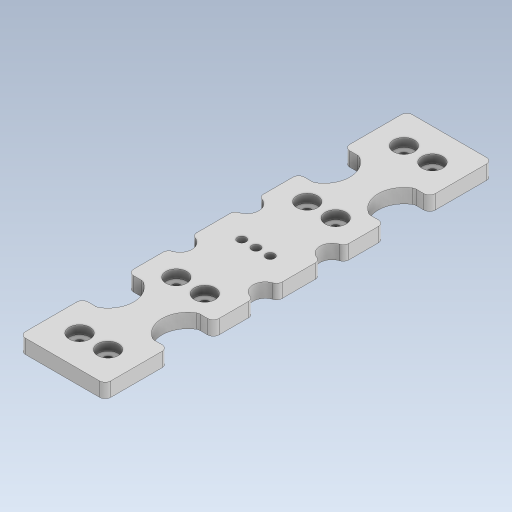
# Autodesk Inventor part: Stopper Lifter
Saved by Autodesk Inventor 2023.5 (Build 275446000, 446)
## iProperties
Created: 2025-10-05
Part Number: Stopper Lifter
Material: Generic
Document SubType Name: Modeling
Designer: Guntur
Density: 1 g/cm^3
Appearance: Default
Author: Guntur
Autodesk Inventor part; units mm, degrees
ref_plane "YZ Plane" through (0, 0, 0) normal (1, 0, 0) x (0, 1, 0)
ref_plane "XZ Plane" through (0, 0, 0) normal (0, 1, 0) x (-1, 0, 0)
ref_plane "XY Plane" through (0, 0, 0) normal (0, 0, 1) x (1, 0, 0)
sketch "Sketch1" plane through (0, 0, 0) normal (0, 1, 0) x (-1, 0, 0)
  line L0 (13.7897, -1.2319) -> (-9.6368, -1.2319) construction
  line L1 (0.7897, 10.3965) -> (0.7897, -17.2319) construction
  line L2 (0.7897, -1.2319) -> (15.7897, -1.2319)
  line L3 (15.7897, -1.2319) -> (15.7897, -7.0606)
  line L4 (15.7897, -8.7319) -> (0.7897, -8.7319)
  line L5 (0.7897, -8.7319) -> (0.7897, -1.2319)
  line L6 (21.7897, -1.2319) -> (-22.2103, -1.2319) construction
  line L7 (0.7897, 17.7681) -> (0.7897, -29.2319) construction
  circle A0 centre (5.7897, -24.2319) radius 3.65
  circle A1 centre (5.7897, -24.2319) radius 5
  circle A2 centre (5.7897, -58.2319) radius 3.65
  circle A3 centre (5.7897, -58.2319) radius 5
  line L8 (0.7897, -17.2319) -> (15.7897, -17.2319)
  line L9 (15.7897, -18.9033) -> (15.7897, -29.2319)
  line L10 (13.7897, -31.2319) -> (11.138, -31.2319)
  line L11 (0.7897, -31.2319) -> (0.7897, -17.2319)
  line L12 (0.7897, -51.2319) -> (15.7897, -51.2319)
  line L13 (15.7897, -51.2319) -> (15.7897, -65.2319)
  line L14 (15.7897, -65.2319) -> (0.7897, -65.2319)
  line L15 (0.7897, -65.2319) -> (0.7897, -51.2319)
  arc A4 (14.4297, -8.9554) -> (14.4297, -17.0085) centre (15.7897, -12.9819) ccw
  line L16 (15.7897, -51.2319) -> (0.7897, -51.2319)
  line L17 (0.7897, -51.2319) -> (0.7897, -47.2319)
  line L18 (11.138, -47.2319) -> (13.7897, -47.2319)
  line L19 (15.7897, -49.2319) -> (15.7897, -51.2319)
  line L20 (15.7897, -65.2319) -> (0.7897, -65.2319)
  line L21 (0.7897, -65.2319) -> (0.7897, -69.2319)
  line L22 (0.7897, -69.2319) -> (13.7897, -69.2319)
  line L23 (15.7897, -67.2319) -> (15.7897, -65.2319)
  arc A5 (14.4297, -8.9554) -> (15.7897, -7.0606) centre (13.7897, -7.0606) ccw
  arc A6 (15.7897, -18.9033) -> (14.4297, -17.0085) centre (13.7897, -18.9033) ccw
  arc A7 (-12.8503, -17.0085) -> (-14.2103, -18.9033) centre (-12.2103, -18.9033) ccw
  circle A8 centre (-4.2103, -24.2319) radius 3.65
  circle A9 centre (-4.2103, -24.2319) radius 5
  line L24 (0.7897, -17.2319) -> (-14.2103, -17.2319)
  arc A10 (-12.8503, -17.0085) -> (-12.8503, -8.9554) centre (-14.2103, -12.9819) ccw
  arc A11 (-14.2103, -7.0606) -> (-12.8503, -8.9554) centre (-12.2103, -7.0606) ccw
  line L25 (-14.2103, -8.7319) -> (0.7897, -8.7319)
  line L26 (-14.2103, -1.2319) -> (-14.2103, -7.0606)
  line L27 (-14.2103, -18.9033) -> (-14.2103, -29.2319)
  line L28 (-12.2103, -31.2319) -> (-9.5586, -31.2319)
  line L29 (-14.2103, -49.2319) -> (-14.2103, -51.2319)
  line L30 (-9.5586, -47.2319) -> (-12.2103, -47.2319)
  line L31 (0.7897, -51.2319) -> (-14.2103, -51.2319)
  line L32 (-14.2103, -51.2319) -> (0.7897, -51.2319)
  line L33 (-14.2103, -51.2319) -> (-14.2103, -65.2319)
  circle A12 centre (-4.2103, -58.2319) radius 3.65
  circle A13 centre (-4.2103, -58.2319) radius 5
  line L34 (-14.2103, -67.2319) -> (-14.2103, -65.2319)
  line L35 (-14.2103, -65.2319) -> (0.7897, -65.2319)
  line L36 (-14.2103, -65.2319) -> (0.7897, -65.2319)
  line L37 (0.7897, -69.2319) -> (-12.2103, -69.2319)
  line L38 (0.7897, 6.2681) -> (0.7897, -1.2319)
  arc A14 (-12.8503, 6.4915) -> (-12.8503, 14.5446) centre (-14.2103, 10.5181) ccw
  line L39 (-14.2103, 6.2681) -> (0.7897, 6.2681)
  line L40 (-14.2103, -1.2319) -> (-14.2103, 4.5967)
  arc A15 (-12.8503, 6.4915) -> (-14.2103, 4.5967) centre (-12.2103, 4.5967) ccw
  line L41 (15.7897, -1.2319) -> (15.7897, 4.5967)
  line L42 (15.7897, 6.2681) -> (0.7897, 6.2681)
  line L43 (0.7897, -12.8604) -> (0.7897, 14.7681) construction
  line L44 (0.7897, -20.2319) -> (0.7897, 26.7681) construction
  circle A16 centre (5.7897, 55.7681) radius 3.65
  circle A17 centre (5.7897, 55.7681) radius 5
  line L45 (0.7897, 48.7681) -> (15.7897, 48.7681)
  line L46 (15.7897, 48.7681) -> (15.7897, 62.7681)
  line L47 (15.7897, 62.7681) -> (0.7897, 62.7681)
  line L48 (0.7897, 62.7681) -> (0.7897, 48.7681)
  line L49 (15.7897, 48.7681) -> (0.7897, 48.7681)
  line L50 (11.138, 44.7681) -> (13.7897, 44.7681)
  line L51 (15.7897, 45.7681) -> (15.7897, 48.7681)
  line L52 (15.7897, 62.7681) -> (0.7897, 62.7681)
  line L53 (0.7897, 66.7681) -> (13.7897, 66.7681)
  line L54 (15.7897, 64.7681) -> (15.7897, 62.7681)
  line L55 (0.7897, 62.7681) -> (0.7897, 66.7681)
  line L56 (13.7897, 28.7681) -> (11.138, 28.7681)
  circle A18 centre (5.7897, 21.7681) radius 3.65
  circle A19 centre (5.7897, 21.7681) radius 5
  line L57 (0.7897, 14.7681) -> (15.7897, 14.7681)
  line L58 (15.7897, 16.4394) -> (15.7897, 27.7681)
  arc A20 (14.4297, 14.5446) -> (14.4297, 6.4915) centre (15.7897, 10.5181) ccw
  arc A21 (15.7897, 4.5967) -> (14.4297, 6.4915) centre (13.7897, 4.5967) ccw
  arc A22 (14.4297, 14.5446) -> (15.7897, 16.4394) centre (13.7897, 16.4394) ccw
  line L59 (0.7897, 14.7681) -> (-14.2103, 14.7681)
  arc A23 (-14.2103, 16.4394) -> (-12.8503, 14.5446) centre (-12.2103, 16.4394) ccw
  circle A24 centre (-4.2103, 21.7681) radius 3.65
  line L60 (-14.2103, 16.4394) -> (-14.2103, 26.7681)
  line L61 (-12.2103, 28.7681) -> (-9.5586, 28.7681)
  line L62 (0.7897, 28.7681) -> (0.7897, 14.7681)
  circle A25 centre (-4.2103, 21.7681) radius 5
  line L63 (0.7897, 66.7681) -> (-12.2103, 66.7681)
  line L64 (-14.2103, 64.7681) -> (-14.2103, 62.7681)
  line L65 (0.7897, 48.7681) -> (0.7897, 44.7681)
  circle A26 centre (-4.2103, 55.7681) radius 3.65
  line L66 (-14.2103, 62.7681) -> (0.7897, 62.7681)
  line L67 (-14.2103, 62.7681) -> (0.7897, 62.7681)
  line L68 (-14.2103, 48.7681) -> (-14.2103, 62.7681)
  line L69 (0.7897, 48.7681) -> (-14.2103, 48.7681)
  line L70 (-14.2103, 48.7681) -> (0.7897, 48.7681)
  line L71 (-14.2103, 46.7681) -> (-14.2103, 48.7681)
  line L72 (-9.5586, 44.7681) -> (-12.2103, 44.7681)
  circle A27 centre (-4.2103, 55.7681) radius 5
  arc A28 (15.7897, 64.7681) -> (13.7897, 66.7681) centre (13.7897, 64.7681) ccw
  arc A29 (-12.2103, 66.7681) -> (-14.2103, 64.7681) centre (-12.2103, 64.7681) ccw
  arc A30 (13.7897, -69.2319) -> (15.7897, -67.2319) centre (13.7897, -67.2319) ccw
  arc A31 (-14.2103, -67.2319) -> (-12.2103, -69.2319) centre (-12.2103, -67.2319) ccw
  arc A32 (10.0879, 44.4702) -> (10.0879, 29.0659) centre (14.8397, 36.7681) ccw
  line L73 (15.7897, 46.7681) -> (15.7897, 45.7681)
  line L74 (15.7897, 26.7681) -> (15.7897, 27.7681)
  arc A33 (13.7897, 44.7681) -> (15.7897, 46.7681) centre (13.7897, 46.7681) ccw
  arc A34 (11.138, 44.7681) -> (10.0879, 44.4702) centre (11.138, 42.7681) ccw
  arc A35 (10.0879, 29.0659) -> (11.138, 28.7681) centre (11.138, 30.7681) ccw
  arc A36 (15.7897, 26.7681) -> (13.7897, 28.7681) centre (13.7897, 26.7681) ccw
  arc A37 (-8.5085, 29.0659) -> (-8.5085, 44.4702) centre (-13.2603, 36.7681) ccw
  line L75 (-14.2103, 45.7681) -> (-14.2103, 44.7681)
  line L76 (-14.2103, 27.7681) -> (-14.2103, 28.7681)
  arc A38 (-8.5085, 44.4702) -> (-9.5586, 44.7681) centre (-9.5586, 42.7681) ccw
  arc A39 (-9.5586, 28.7681) -> (-8.5085, 29.0659) centre (-9.5586, 30.7681) ccw
  arc A40 (-12.2103, 28.7681) -> (-14.2103, 26.7681) centre (-12.2103, 26.7681) ccw
  arc A41 (-14.2103, 46.7681) -> (-12.2103, 44.7681) centre (-12.2103, 46.7681) ccw
  arc A42 (10.0879, -31.5298) -> (10.0879, -46.9341) centre (14.8397, -39.2319) ccw
  arc A43 (-8.5085, -46.9341) -> (-8.5085, -31.5298) centre (-13.2603, -39.2319) ccw
  line L77 (-14.2103, -30.2319) -> (-14.2103, -31.2319)
  line L78 (-14.2103, -47.2319) -> (-14.2103, -48.2319)
  line L79 (15.7897, -30.2319) -> (15.7897, -31.2319)
  line L80 (15.7897, -47.2319) -> (15.7897, -48.2319)
  arc A44 (13.7897, -31.2319) -> (15.7897, -29.2319) centre (13.7897, -29.2319) ccw
  arc A45 (15.7897, -49.2319) -> (13.7897, -47.2319) centre (13.7897, -49.2319) ccw
  arc A46 (10.0879, -46.9341) -> (11.138, -47.2319) centre (11.138, -45.2319) ccw
  arc A47 (11.138, -31.2319) -> (10.0879, -31.5298) centre (11.138, -33.2319) ccw
  arc A48 (-9.5586, -47.2319) -> (-8.5085, -46.9341) centre (-9.5586, -45.2319) ccw
  arc A49 (-12.2103, -47.2319) -> (-14.2103, -49.2319) centre (-12.2103, -49.2319) ccw
  arc A50 (-8.5085, -31.5298) -> (-9.5586, -31.2319) centre (-9.5586, -33.2319) ccw
  arc A51 (-14.2103, -29.2319) -> (-12.2103, -31.2319) centre (-12.2103, -29.2319) ccw
  circle A52 centre (5.7897, 55.7681) radius 1.5
  circle A53 centre (-4.2103, 55.7681) radius 1.5
  circle A54 centre (5.7897, 21.7681) radius 1.5
  circle A55 centre (-4.2103, 21.7681) radius 1.5
  circle A56 centre (5.7897, -24.2319) radius 1.5
  circle A57 centre (-4.2103, -24.2319) radius 1.5
  circle A58 centre (5.7897, -58.2319) radius 1.5
  circle A59 centre (-4.2103, -58.2319) radius 1.5
  circle A60 centre (0.7897, -1.2319) radius 1.5
  circle A61 centre (5.7897, -1.2319) radius 1.5
  circle A62 centre (-4.2103, -1.2319) radius 1.5
  point P0 (0, 0)
  point P1 (15.7897, -69.2319)
  point P2 (-14.2103, -69.2319)
  point P3 (15.7897, 44.7681)
  point P4 (15.7897, 66.7681)
  point P5 (15.7897, 28.7681)
  point P6 (-14.2103, 66.7681)
  point P7 (10.6085, 44.7681)
  point P8 (10.6085, 28.7681)
  point P9 (-9.0292, 28.7681)
  point P10 (-9.0292, 44.7681)
  point P11 (10.6085, -31.2319)
  point P12 (10.6085, -47.2319)
  point P13 (-9.0292, -31.2319)
  point P14 (-9.0292, -47.2319)
  dimension "d0" = 15
  dimension "d1" = 7.5
  dimension "d2" = 7.3
  dimension "d3" = 23
  dimension "d4" = 10
  dimension "d5" = 7.3
  dimension "d6" = 10
  dimension "d7" = 34
  dimension "d8" = 4
  dimension "d9" = 4
  dimension "d10" = 2
  dimension "d11" = 2
  dimension "d12" = 2
  dimension "d13" = 2
  dimension "d14" = 2
  dimension "d19" = 3
  dimension "d20" = 3
  dimension "d21" = 3
  dimension "d22" = 3
  dimension "d23" = 3
  dimension "d24" = 3
  dimension "d25" = 3
  dimension "d26" = 3
  dimension "d27" = 3
  dimension "d28" = 3
  dimension "d29" = 3
  constraints: 162 end point, 88 point on circle, 73 symmetric about line, 68 point on line, 63 centre point, 46 tangent, 18 coincident, 17 equal radius, 11 parallel, 7 horizontal, 6 vertical, 5 perpendicular, 4 collinear, 22 other
  measures "d0" distance of L4.start L5.start
  measures "d1" distance of L2.end L4.start
  measures "d2" diameter of A0
  measures "d3" distance from line of L2 A0.centre
  measures "d4" diameter of A1
  measures "d5" diameter of A2
  measures "d6" diameter of A3
  measures "d7" distance of A3.centre A0.centre
  measures "d8" distance of L17.start L17.end
  measures "d9" distance of L22.start L20.end
  measures "d10" radius of A5
  measures "d11" radius of A28
  measures "d12" radius of A33
  measures "d13" radius of A38
  measures "d14" radius of A44
  measures "d19" diameter of A52
  measures "d20" diameter of A53
  measures "d21" diameter of A54
  measures "d22" diameter of A55
  measures "d23" diameter of A56
  measures "d24" diameter of A57
  measures "d25" diameter of A58
  measures "d26" diameter of A59
  measures "d27" diameter of A60
  measures "d28" diameter of A61
  measures "d29" diameter of A62
extrude "Extrusion1" add sketch "Sketch1" along normal blind 5 contours A60 L38 L42 A21 L41 L2 A61 | L2 A61 L3 A5 L4 L5 A60 | L5 L25 A11 L26 L40 A15 L39 L38 A60 | L4 A5 A4 A6 L8 L24 A7 A10 A11 L25 | L39 A15 A14 A23 L59 L57 A22 A20 A21 L42 | A6 L9 A44 L10 A47 A42 A46 L18 A45 L19 L12 L31 L29 A49 L30 A48 A43 A50 L28 A51 L27 A7 L24 L8 | A23 L60 A40 L61 A39 A37 A38 L72 A41 L71 L69 L45 L51 A33 L50 A34 A32 A35 L56 A36 L58 A22 L57 L59 | A3 | L13 L14 L15 L12 | A13 | L31 L15 L35 L33 | A27 | L68 L66 L48 L69 | A17 | L45 L48 L47 L46 | L23 A30 L22 L21 L14 | L35 L21 L37 A31 L34 | L64 A29 L63 L55 L66 | L47 L55 L53 A28 L54 | A1 | A9 | A19 | A25
extrude "Extrusion2" add sketch "Sketch1" along normal blind 2 contours A0 | A2 | A8 | A12 | A16 | A18 | A24 | A26
body "Solid1"
